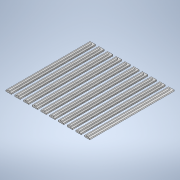
# Autodesk Inventor part: structure2
Saved by Autodesk Inventor 2022 (Build 260153000, 153)
## iProperties
Created: 2022-04-07
Part Number: structure2
Material: Generic
Document SubType Name: Modeling
Designer: ten26
Density: 1 g/cm^3
Appearance: Default
Author: ten26
Autodesk Inventor part; units mm, degrees
ref_plane "YZ Plane" through (0, 0, 0) normal (1, 0, 0) x (0, 1, 0)
ref_plane "XZ Plane" through (0, 0, 0) normal (0, 1, 0) x (-1, 0, 0)
ref_plane "XY Plane" through (0, 0, 0) normal (0, 0, 1) x (1, 0, 0)
sketch "Sketch1" plane through (0, 0, 0) normal (0, 1, 0) x (-1, 0, 0)
  line L0 (2.65, -41) -> (-2.65, -41)
  line L1 (-2.65, -41) -> (-2.65, 41)
  line L2 (-2.65, 41) -> (2.65, 41)
  line L3 (2.65, 41) -> (2.65, -41)
  line L4 (2.65, -41) -> (-2.65, 41) construction
  line L5 (-2.65, -41) -> (2.65, 41) construction
  line L6 (-1.2752, 41) -> (1.1507, 41)
  line L7 (1.1507, 41) -> (1.1507, 41)
  line L8 (1.1507, 41) -> (-1.2752, 41)
  line L9 (-1.2752, 41) -> (-1.2752, 41)
  point P0 (0, 0)
  dimension "d0" = 5.3
  dimension "d1" = 82
  constraints: 20 end point, 4 equal length, 2 horizontal, 2 midpoint, 2 perpendicular, 2 point on line
  measures "d0" distance of L1.end L2.end
  measures "d1" distance of L0.end L1.end
extrude "Extrusion1" add sketch "Sketch1" along normal blind 1.1
sketch "Sketch2" plane through (0, 1.1, 0) normal (0, 1, 0) x (1, 0, 0)
  line L0 (-2.65, -41) -> (2.65, -41) projected
  line L1 (0.8, -41) -> (-0.8, -41)
  line L2 (-0.8, -41) -> (-0.8, 39)
  line L3 (-0.8, 39) -> (0.8, 39)
  line L4 (0.8, 39) -> (0.8, -41)
  line L5 (2.65, -41) -> (2.65, 41) projected
  line L6 (-2.65, 41) -> (-2.65, -41) projected
  point P0 (0, 0)
  dimension "d4" = 80
  dimension "d5" = 1.6
  dimension "d6" = 5.3
  dimension "d7" = 1.85
  constraints: 8 end point, 2 parallel, 1 horizontal, 1 perpendicular, 1 point on line
  measures "d4" distance between parallel lines of L0 L3
  measures "d5" distance between parallel lines of L4 L2
  measures "d6" distance between parallel lines of L5 L6
  measures "d7" distance between parallel lines of L2 L6
extrude "Extrusion2" add sketch "Sketch2" along normal blind 1
pattern_linear "Rectangular Pattern1" count 10 spacing 8.5 along (1, 0, 0) of "Extrusion1", "Extrusion2"
equation "\"d7\" = 0.5 * d6 - 0.5 * d5"
equation "\"base_add\" = 0.6"
body "Solid1"
